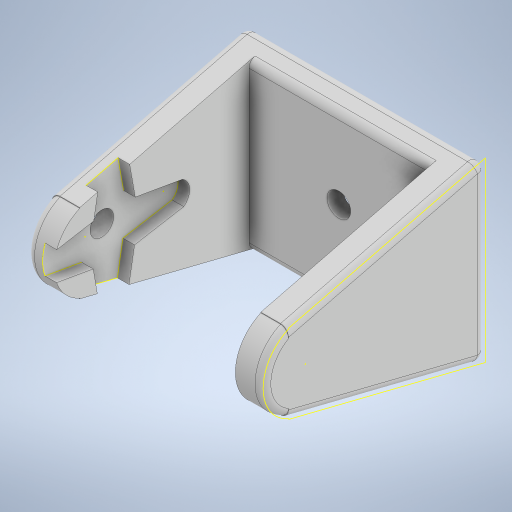
# Autodesk Inventor part: schouder(s)
Saved by Autodesk Inventor 2023 (Build 270158000, 158)
## iProperties
Created: 2022-04-21
Part Number: schouder(s)
Material: Generic
Document SubType Name: Modeling
Designer: kajve
Density: 1 g/cm^3
Appearance: Default
Author: kajve
## iProperties of the stored document schouder(s)_3DPrint.ipt
Created: 2022-05-23
Part Number: schouder(s)_3DPrint
Material: Generic
Document SubType Name: Modeling
Designer: kajve
Density: 1 g/cm^3
Appearance: Default
Author: kajve
Autodesk Inventor part; units mm, degrees
ref_plane "YZ Plane" through (0, 0, 0) normal (1, 0, 0) x (0, 1, 0)
ref_plane "XZ Plane" through (0, 0, 0) normal (0, 1, 0) x (-1, 0, 0)
ref_plane "XY Plane" through (0, 0, 0) normal (0, 0, 1) x (1, 0, 0)
sketch "Sketch1" plane through (0, 0, 0) normal (0, 0, 1) x (1, 0, 0)
  point P0 (0, 0)
sketch "Sketch2" plane through (0, 0, 0) normal (0, 0, 1) x (1, 0, 0)
  line L0 (0, 0) -> (60, 0)
  line L1 (60, 0) -> (60, 45)
  line L2 (60, 45) -> (0, 45)
  line L3 (0, 45) -> (0, 0)
  dimension "d0" = 60
  dimension "d1" = 45
  constraints: 8 end point, 2 parallel, 1 horizontal, 1 perpendicular
  measures "d0" distance of L2.end L1.end
  measures "d1" distance of L1.end L0.end
extrude "Extrusion1" add sketch "Sketch2" along normal blind 50
sketch "Sketch3" plane through (60, 0, 0) normal (1, 0, 0) x (0, 0, -1)
  line L0 (0, 45) -> (-50, 45) projected
  line L1 (-50, 0) -> (-50, 45) projected
  line L2 (0, 0) -> (-50, 0) projected
  line L3 (0, 45) -> (-50, 32.5336)
  line L4 (0, 45) -> (51.5307, 45) construction
  line L5 (0, 0) -> (-50, 12.4664)
  line L6 (0, 0) -> (51.5307, 0) construction
  dimension "d4" = 166
  dimension "d5" = 166
  constraints: 8 end point, 2 equal length, 2 horizontal, 2 point on line
  measures "d4" angle of L3 L4
  measures "d5" angle of L6 L5
extrude "Extrusion2" cut sketch "Sketch3" against normal through all
sketch "Sketch4" plane through (60, 0, 0) normal (1, 0, 0) x (0, 0, -1)
  line L0 (-50, 12.4664) -> (-50, 32.5336) projected
  circle A0 centre (-45.6937, 22.5) radius 10.7721
  point P0 (-50, 32.3739)
  point P1 (-50, 12.6261)
  constraints: 1 centre point
extrude "Extrusion3" add sketch "Sketch4" against normal blind 60 contours A0 L0 picked at (-52.7772, 22.9072)
sketch "Sketch6" plane through (0, 0, 0) normal (0, 0, -1) x (-1, 0, 0)
  line L0 (0, 0) -> (-60, 0) projected
  line L1 (-60, 45) -> (0, 45) projected
  line L2 (-7, 0) -> (-53, 0)
  line L3 (-53, 0) -> (-53, 45)
  line L4 (-53, 45) -> (-7, 45)
  line L5 (-7, 45) -> (-7, 0)
  point P0 (-7, 45)
  dimension "d10" = 46
  constraints: 8 end point, 2 parallel, 2 point on line, 1 horizontal, 1 perpendicular
  measures "d10" distance of L3.end L4.end
extrude "Extrusion4" cut sketch "Sketch6" against normal through all
sketch "Sketch7" plane through (0, 0, 0) normal (0, 0, -1) x (-1, 0, 0)
  line L0 (-7, 45) -> (-7, 0) projected
  line L1 (-7, 32.5336) -> (-7, 45) projected
  line L2 (-53, 0) -> (-60, 0) projected
  line L3 (-7, 45) -> (-53, 45)
  line L4 (-53, 45) -> (-53, 0)
  line L5 (-53, 0) -> (-7, 0)
  line L6 (-7, 0) -> (-7, 45)
  point P0 (-7, 0)
  constraints: 8 end point, 2 parallel, 1 horizontal, 1 perpendicular
extrude "Extrusion5" add sketch "Sketch7" against normal blind 7
sketch "Sketch8" plane through (60, 0, 0) normal (1, 0, 0) x (0, 0, -1)
  line L0 (0, 45) -> (-50, 32.5336) projected
  line L1 (-50, 32.3739) -> (-50, 32.5336) projected
  arc A0 (-50, 32.3739) -> (-50, 12.6261) centre (-45.6937, 22.5) ccw projected
  line L2 (-50, 12.4664) -> (-50, 12.6261) projected
  line L3 (-50, 12.4664) -> (0, 0) projected
  line L4 (0, 0) -> (0, 45) projected
sketch "Sketch9" plane through (53, 43.2547, 7) normal (1, 0, 0) x (0, 0, -1)
  line L0 (7, 1.7453) -> (0, 0) projected
  line L1 (7, 1.7453) -> (0, 1.7453) projected
  line L2 (0, 0) -> (0, 1.7453) projected
  line L3 (7, -43.2547) -> (7, 1.7453) projected
  line L4 (0, 0) -> (7, 1.7453)
  line L5 (7, 1.7453) -> (0, 1.7453)
  constraints: 4 end point, 1 collinear
extrude "Extrusion6" cut sketch "Sketch9" against normal through all
sketch "Sketch10" plane through (53, 0, 7) normal (1, 0, 0) x (0, 0, -1)
  line L0 (0, 1.7453) -> (7, 0) projected
  line L1 (0, 0) -> (0, 1.7453) projected
  line L2 (7, 0) -> (0, 0) projected
  line L3 (-43, 12.4664) -> (7, 0) projected
  line L4 (0, 43.2547) -> (0, 1.7453) projected
  line L5 (7, 0) -> (0, 1.7453)
  line L6 (0, 1.7453) -> (0, 0)
  constraints: 4 end point, 1 collinear
extrude "Extrusion7" cut sketch "Sketch10" against normal through all
fillet "Fillet1" radius 2 12 edges at (60, 6.2332, 25) (60, 22.5, 56.4658) (60, 38.7668, 25) (60, 22.5, 0) (30, 0, 0) (30, 45, 0) (0, 22.5, 0) (0, 6.2332, 25) (0, 22.5, 56.4658) (0, 38.7668, 25) (30, 43.2547, 7) (30, 1.7453, 7)
sketch "Sketch11" plane through (0, 0, 0) normal (0, 0, -1) x (-1, 0, 0)
  arc A0 (-46.6851, 26.0014) -> (-47.1755, 19.6826) centre (-45.4589, 22.7278) ccw
  arc A1 (-33.0497, 5.9023) -> (-26.7251, 5.4079) centre (-29.7704, 7.1528) ccw
  arc A2 (-12.5069, 19.7206) -> (-13.0798, 26.0769) centre (-14.2683, 22.7658) ccw
  arc A3 (-26.4282, 39.3355) -> (-32.8536, 40.0857) centre (-29.8083, 38.2761) ccw
  line L0 (-46.6851, 26.0014) -> (-34.956, 28.0437)
  line L1 (-34.956, 28.0437) -> (-32.8536, 40.0857)
  line L2 (-26.4282, 39.3355) -> (-24.4165, 28.0327)
  line L3 (-24.4165, 28.0327) -> (-13.0798, 26.0769)
  line L4 (-12.5069, 19.7206) -> (-24.5937, 17.616)
  line L5 (-24.5937, 17.616) -> (-26.7251, 5.4079)
  line L6 (-33.0497, 5.9023) -> (-35.0882, 17.5779)
  line L7 (-47.1755, 19.6826) -> (-35.0882, 17.5779)
  line L8 (-58, 42.4401) -> (-2, 42.4401) projected
  line L9 (-2, 2.5599) -> (-58, 2.5599) projected
  line L10 (-30, 42.4401) -> (-30, 2.5599) construction
  line L11 (-53, 3.3079) -> (-7, 3.3079) construction
  line L12 (-58, 32.3739) -> (-58, 12.6261) construction
  line L13 (-58, 22.5) -> (-2, 22.5) construction
  line L14 (-2, 42.4401) -> (-2, 2.5599) construction
  constraints: 20 end point, 8 point on circle, 4 centre point, 4 midpoint, 1 perpendicular
extrude "Extrusion8" cut sketch "Sketch11" against normal blind 3
sketch "Sketch12" plane through (7, 22.5, 45.6937) normal (1, 0, 0) x (0, 0, -1)
  line L0 (-4.3063, 10.0336) -> (40.2099, 21.1327) projected
  arc A0 (-4.3063, 9.8739) -> (-4.3063, -9.8739) centre (0, 0) ccw projected
  line L1 (40.2099, -21.1327) -> (-4.3063, -10.0336) projected
  line L2 (38.6937, -19.1921) -> (38.6937, 19.1921)
  arc A1 (40.2099, 21.1327) -> (38.6937, 19.1921) centre (40.6937, 19.1921) ccw
  line L3 (-4.3063, 10.0336) -> (40.2099, 21.1327)
  line L4 (-4.3063, 9.8739) -> (-4.3063, 10.0336)
  arc A2 (-4.3063, 9.8739) -> (-4.3063, -9.8739) centre (0, 0) ccw
  line L5 (-4.3063, -10.0336) -> (-4.3063, -9.8739)
  line L6 (40.2099, -21.1327) -> (-4.3063, -10.0336)
  arc A3 (38.6937, -19.1921) -> (40.2099, -21.1327) centre (40.6937, -19.1921) ccw
  arc A4 (-12.4398, 3.268) -> (-12.9526, -3.0638) centre (-11.2621, -0.014) ccw
  arc A5 (1.0385, -16.2174) -> (7.5066, -17.1336) centre (4.4264, -15.5891) ccw
  arc A6 (22.096, -2.9505) -> (21.7404, 3.2275) centre (19.9285, 0.024) ccw
  arc A7 (7.5788, 17.6601) -> (1.4591, 18.0075) centre (4.3884, 15.5342) ccw
  line L7 (-12.4398, 3.268) -> (-0.7592, 5.3019)
  line L8 (-0.7592, 5.3019) -> (1.4591, 18.0075)
  line L9 (7.5788, 17.6601) -> (9.7803, 5.2908)
  line L10 (9.7803, 5.2908) -> (21.7404, 3.2275)
  line L11 (22.096, -2.9505) -> (9.6031, -5.1258)
  line L12 (9.6031, -5.1258) -> (7.5066, -17.1336)
  line L13 (1.0385, -16.2174) -> (-0.8914, -5.1639)
  line L14 (-12.9526, -3.0638) -> (-0.8914, -5.1639)
  line L15 (38.6937, -19.1921) -> (38.6937, 19.1921) projected
  arc A8 (40.2099, 21.1327) -> (38.6937, 19.1921) centre (40.6937, 19.1921) ccw projected
  line L16 (-4.3063, 10.0336) -> (40.2099, 21.1327) projected
  line L17 (-4.3063, 9.8739) -> (-4.3063, 10.0336) projected
  arc A9 (-4.3063, 9.8739) -> (-4.3063, -9.8739) centre (0, 0) ccw projected
  line L18 (-4.3063, -10.0336) -> (-4.3063, -9.8739) projected
  line L19 (40.2099, -21.1327) -> (-4.3063, -10.0336) projected
  arc A10 (38.6937, -19.1921) -> (40.2099, -21.1327) centre (40.6937, -19.1921) ccw projected
  arc A11 (-4.3063, 9.8739) -> (-4.3063, -9.8739) centre (0, 0) ccw projected
  line L20 (-4.3063, 9.8739) -> (-4.3063, 10.0336) projected
  line L21 (-4.3063, 10.0336) -> (40.2099, 21.1327) projected
  line L22 (40.2099, 21.1327) -> (43.2099, 21.8807) projected
  arc A12 (45.6937, 19.9401) -> (43.2099, 21.8807) centre (43.6937, 19.9401) ccw projected
  line L23 (45.6937, 19.9401) -> (45.6937, -19.9401) projected
  arc A13 (43.2099, -21.8807) -> (45.6937, -19.9401) centre (43.6937, -19.9401) ccw projected
  line L24 (43.2099, -21.8807) -> (40.2099, -21.1327) projected
  line L25 (40.2099, -21.1327) -> (-4.3063, -10.0336) projected
  line L26 (-4.3063, -10.0336) -> (-4.3063, -9.8739) projected
  arc A14 (40.2099, 21.1327) -> (38.6937, 19.1921) centre (40.6937, 19.1921) ccw projected
  line L27 (38.6937, -19.1921) -> (38.6937, 19.1921) projected
  arc A15 (38.6937, -19.1921) -> (40.2099, -21.1327) centre (40.6937, -19.1921) ccw projected
  point P0 (45.6937, -22.5)
  point P1 (45.6937, -22.5)
  point P2 (8.3735, 13.195)
  point P3 (0.2659, 11.1736)
  point P4 (-10.1274, 3.6706)
  point P5 (-10.171, -3.5481)
  point P6 (0.1529, -11.1454)
  point P7 (8.2018, -13.1522)
  constraints: 26 end point, 14 point on circle, 7 centre point
extrude "Extrusion9" cut sketch "Sketch12" against normal blind 3 contours L0 L9 L10 A6 L11 L12 L1 L13 L14 A0 L7 L8
sketch "Sketch13" plane through (0, 0, 3) normal (0, 0, -1) x (-1, 0, 0)
  circle A0 centre (-29.8083, 23.0816) radius 3
  point P0 (0, 0)
  dimension "d25" = 6
  constraints: 1 centre point
  measures "d25" diameter of A0
sketch "Sketch14" plane through (4, 22.5, 45.6937) normal (1, 0, 0) x (0, 0, -1)
  arc A0 (22.096, -2.9505) -> (21.7404, 3.2275) centre (19.9285, 0.024) ccw projected
  line L0 (9.7803, 5.2908) -> (21.7404, 3.2275) projected
  line L1 (8.3735, 13.195) -> (9.7803, 5.2908) projected
  line L2 (0.2659, 11.1736) -> (8.3735, 13.195) projected
  line L3 (-0.7592, 5.3019) -> (0.2659, 11.1736) projected
  line L4 (-10.1274, 3.6706) -> (-0.7592, 5.3019) projected
  arc A1 (-10.1274, 3.6706) -> (-10.171, -3.5481) centre (0, 0) ccw projected
  line L5 (-0.8914, -5.1639) -> (-10.171, -3.5481) projected
  line L6 (0.1529, -11.1454) -> (-0.8914, -5.1639) projected
  line L7 (8.2018, -13.1522) -> (0.1529, -11.1454) projected
  line L8 (9.6031, -5.1258) -> (8.2018, -13.1522) projected
  line L9 (22.096, -2.9505) -> (9.6031, -5.1258) projected
  point P0 (45.6937, -22.5)
extrude "Extrusion10" cut sketch "Sketch13" against normal blind 10
sketch "Sketch15" plane through (4, 22.5, 45.6937) normal (1, 0, 0) x (0, 0, -1)
  line L0 (0.2659, 11.1736) -> (8.3735, 13.195) projected
  line L1 (8.2018, -13.1522) -> (0.1529, -11.1454) projected
  line L2 (9.6031, -5.1258) -> (8.2018, -13.1522) construction
  arc A0 (22.096, -2.9505) -> (21.7404, 3.2275) centre (19.9285, 0.024) ccw projected
  line L3 (9.7803, 5.2908) -> (21.7404, 3.2275) projected
  line L4 (8.3735, 13.195) -> (9.7803, 5.2908) projected
  line L5 (0.2659, 11.1736) -> (8.3735, 13.195) projected
  line L6 (-0.7592, 5.3019) -> (0.2659, 11.1736) projected
  line L7 (-10.1274, 3.6706) -> (-0.7592, 5.3019) projected
  arc A1 (-10.1274, 3.6706) -> (-10.171, -3.5481) centre (0, 0) ccw projected
  line L8 (-0.8914, -5.1639) -> (-10.171, -3.5481) projected
  line L9 (0.1529, -11.1454) -> (-0.8914, -5.1639) projected
  line L10 (8.2018, -13.1522) -> (0.1529, -11.1454) projected
  line L11 (9.6031, -5.1258) -> (8.2018, -13.1522) projected
  line L12 (22.096, -2.9505) -> (9.6031, -5.1258) projected
  arc A2 (22.096, -2.9505) -> (21.7404, 3.2275) centre (19.9285, 0.024) ccw projected
  line L13 (9.7803, 5.2908) -> (21.7404, 3.2275) projected
  line L14 (8.3735, 13.195) -> (9.7803, 5.2908) projected
  line L15 (0.2659, 11.1736) -> (8.3735, 13.195) projected
  line L16 (-0.7592, 5.3019) -> (0.2659, 11.1736) projected
  line L17 (-10.1274, 3.6706) -> (-0.7592, 5.3019) projected
  arc A3 (-10.1274, 3.6706) -> (-10.171, -3.5481) centre (0, 0) ccw projected
  line L18 (-0.8914, -5.1639) -> (-10.171, -3.5481) projected
  line L19 (0.1529, -11.1454) -> (-0.8914, -5.1639) projected
  line L20 (8.2018, -13.1522) -> (0.1529, -11.1454) projected
  line L21 (9.6031, -5.1258) -> (8.2018, -13.1522) projected
  line L22 (22.096, -2.9505) -> (9.6031, -5.1258) projected
  arc A4 (22.096, -2.9505) -> (21.7404, 3.2275) centre (19.9285, 0.024) ccw projected
  line L23 (9.7803, 5.2908) -> (21.7404, 3.2275) projected
  line L24 (8.3735, 13.195) -> (9.7803, 5.2908) projected
  line L25 (0.2659, 11.1736) -> (8.3735, 13.195) projected
  line L26 (-0.7592, 5.3019) -> (0.2659, 11.1736) projected
  line L27 (-10.1274, 3.6706) -> (-0.7592, 5.3019) projected
  arc A5 (-10.1274, 3.6706) -> (-10.171, -3.5481) centre (0, 0) ccw projected
  line L28 (-0.8914, -5.1639) -> (-10.171, -3.5481) projected
  line L29 (0.1529, -11.1454) -> (-0.8914, -5.1639) projected
  line L30 (8.2018, -13.1522) -> (0.1529, -11.1454) projected
  line L31 (9.6031, -5.1258) -> (8.2018, -13.1522) projected
  line L32 (22.096, -2.9505) -> (9.6031, -5.1258) projected
  arc A6 (22.096, -2.9505) -> (21.7404, 3.2275) centre (19.9285, 0.024) ccw construction
  line L33 (9.7803, 5.2908) -> (21.7404, 3.2275) construction
  line L34 (8.3735, 13.195) -> (9.7803, 5.2908) construction
  line L35 (0.2659, 11.1736) -> (8.3735, 13.195) construction
  line L36 (-0.7592, 5.3019) -> (0.2659, 11.1736) construction
  line L37 (-10.1274, 3.6706) -> (-0.7592, 5.3019) construction
  arc A7 (-10.1274, 3.6706) -> (-10.171, -3.5481) centre (0, 0) ccw construction
  line L38 (-0.8914, -5.1639) -> (-10.171, -3.5481) construction
  line L39 (0.1529, -11.1454) -> (-0.8914, -5.1639) construction
  line L40 (8.2018, -13.1522) -> (0.1529, -11.1454) construction
  line L41 (9.6031, -5.1258) -> (8.2018, -13.1522) construction
  line L42 (22.096, -2.9505) -> (9.6031, -5.1258) construction
  line L43 (8.3735, 13.195) -> (9.7803, 5.2908) projected
  line L44 (0.1529, -11.1454) -> (-0.8914, -5.1639) projected
  line L45 (9.6031, -5.1258) -> (8.2018, -13.1522) projected
  line L46 (-4.3063, 10.0336) -> (43.2099, 21.8807) projected
  circle A8 centre (4.3019, 0.7365) radius 3
  point P0 (45.6937, -22.5)
  dimension "d29" = 6
  constraints: 1 centre point, 1 coincident, 4 other
  measures "d29" diameter of A8
extrude "Extrusion11" cut sketch "Sketch15" against normal blind 10 contours A8
body "Solid1"
